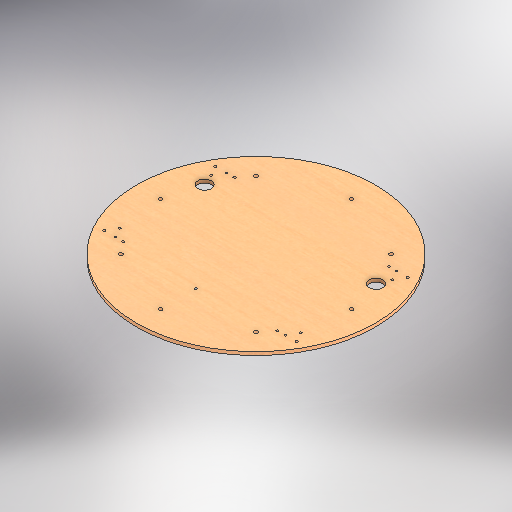
# Autodesk Inventor part: layer3_new
Saved by Autodesk Inventor 2026 (Build 300175050, 175E)
## iProperties
Created: 2025-06-05
Part Number: layer3_new
Material: Generic
Document SubType Name: Modeling
Designer: satom
Density: 1 g/cm^3
Appearance: Default
Author: satom
Autodesk Inventor part; units mm, degrees
ref_plane "YZ Plane" through (0, 0, 0) normal (1, 0, 0) x (0, 1, 0)
ref_plane "XZ Plane" through (0, 0, 0) normal (0, 1, 0) x (-1, 0, 0)
ref_plane "XY Plane" through (0, 0, 0) normal (0, 0, 1) x (1, 0, 0)
sketch "Sketch1" plane through (0, 0, 0) normal (0, 1, 0) x (-1, 0, 0)
  circle A0 centre (0, 0) radius 177
  dimension "d0" = 354
  constraints: 1 centre point, 1 coincident
  measures "d0" diameter of A0
extrude "Extrusion1" add sketch "Sketch1" along normal blind 5
sketch "Sketch2" plane through (0, 5, 0) normal (0, 1, 0) x (1, 0, 0)
  circle A0 centre (-114.3, 82.55) radius 1.7
  line L0 (-177, 0) -> (177, 0) construction
  line L1 (0, 177) -> (0, -177) construction
  circle A1 centre (114.3, 82.55) radius 1.7
  circle A2 centre (-114.3, -82.55) radius 1.7
  circle A3 centre (114.3, -82.55) radius 1.7
  point P0 (0, 0)
  dimension "d3" = 3.4
  dimension "d20" = 82.55
  dimension "d21" = 114.3
  dimension "d24" = 228.6
  dimension "d27" = 165.1
  constraints: 4 centre point, 4 end point, 2 horizontal, 2 vertical, 6 other
  measures "d3" diameter of A0
  measures "d20" distance from line of L0 A0.centre
  measures "d21" distance from line of L1 A0.centre
  measures "d24" distance of A0.centre A1.centre
  measures "d27" distance of A0.centre A2.centre
extrude "Level2 Standoffs" cut sketch "Sketch2" against normal through all
sketch "Sketch3" plane through (0, 5, 0) normal (0, 1, 0) x (1, 0, 0)
  circle A0 centre (-127, 50.8) radius 10.16
  circle A1 centre (127, 50.8) radius 10.16
  circle A2 centre (0, 0) radius 177 construction
  line L0 (0, 177) -> (0, -177) construction
  line L1 (177, 0) -> (-177, 0) construction
  circle A3 centre (0, 0) radius 177 construction
  dimension "d32" = 20.32
  dimension "d33" = 20.32
  dimension "d34" = 127
  dimension "d35" = 127
  dimension "d36" = 50.8
  dimension "d37" = 50.8
  constraints: 5 point on circle, 4 end point, 2 centre point, 1 perpendicular, 1 vertical
  measures "d32" diameter of A0
  measures "d33" diameter of A1
  measures "d34" distance from line of L0 A0.centre
  measures "d35" distance from line of L0 A1.centre
  measures "d36" distance from line of L1 A0.centre
  measures "d37" distance from line of L1 A1.centre
extrude "Wires" cut sketch "Sketch3" against normal through all
sketch "Sketch4" plane through (0, 5, 0) normal (0, 1, 0) x (1, 0, 0)
  line L0 (0, 0) -> (153.2865, -88.5) construction
  circle A0 centre (0, 0) radius 177 construction
  line L1 (-177, 0) -> (177, 0) construction
  circle A1 centre (142.288, -82.15) radius 1.7
  line L2 (142.288, -82.15) -> (134.0391, -77.3875) construction
  line L3 (134.0391, -232.1625) -> (134.0391, -55.1625) construction
  circle A2 centre (134.0391, -67.8625) radius 1.7
  line L4 (268.0782, 0) -> (114.7917, -88.5) construction
  circle A3 centre (125.7902, -82.15) radius 1.7
  circle A4 centre (125.7902, 82.15) radius 1.7
  circle A5 centre (142.288, 82.15) radius 1.7
  circle A6 centre (134.0391, 67.8625) radius 1.7
  line L5 (0, 177) -> (0, -177) construction
  circle A7 centre (-142.288, -82.15) radius 1.7
  circle A8 centre (-134.0391, -67.8625) radius 1.7
  circle A9 centre (-125.7902, -82.15) radius 1.7
  circle A10 centre (-125.7902, 82.15) radius 1.7
  circle A11 centre (-142.288, 82.15) radius 1.7
  circle A12 centre (-134.0391, 67.8625) radius 1.7
  dimension "d40" = 30
  dimension "d41" = 12.7
  dimension "d42" = 9.525
  dimension "d45" = 360
  dimension "d49" = 60
  dimension "d65" = 3.4
  constraints: 12 centre point, 12 end point, 6 point on line, 6 symmetric about line, 5 point on circle, 2 coincident, 1 horizontal, 1 vertical, 30 other
  measures "d40" angle of L0 L1
  measures "d41" distance of L0.end L2.start
  measures "d42" distance of L2.start L2.end
  measures "d65" diameter of A1
extrude "Level4 Standoffs" cut sketch "Sketch4" against normal through all
sketch "Sketch5" plane through (0, 5, 0) normal (0, 1, 0) x (1, 0, 0)
  circle A0 centre (0, -141.44) radius 2.667
  circle A1 centre (0, 0) radius 177 construction
  line L0 (0, -177) -> (89.0082, -177) construction
  circle A2 centre (100.0132, -100.0132) radius 2.667
  circle A3 centre (141.44, 0) radius 2.667
  circle A4 centre (100.0132, 100.0132) radius 2.667
  circle A5 centre (0, 141.44) radius 2.667
  circle A6 centre (-100.0132, 100.0132) radius 2.667
  circle A7 centre (-141.44, 0) radius 2.667
  circle A8 centre (-100.0132, -100.0132) radius 2.667
  dimension "d53" = 5.334
  dimension "d54" = 35.56
  dimension "d57" = 360
  constraints: 8 centre point, 2 end point, 2 horizontal, 1 vertical alignment, 18 other
  measures "d53" diameter of A0
  measures "d54" distance from line of L0 A0.centre
extrude "Zip Ties" cut sketch "Sketch5" against normal through all
sketch "Sketch6" plane through (0, 5, 0) normal (0, 1, 0) x (1, 0, 0)
  circle A0 centre (0, -88.9) radius 1.7
  point P0 (0, 0)
  dimension "d61" = 3.4
  dimension "d62" = 88.9
  constraints: 1 centre point
  measures "d61" diameter of A0
  measures "d62" distance of A0.centre point (0, 0)
extrude "Extrusion6" cut sketch "Sketch6" against normal blind 25.4
equation "\"d0\" = robot_diameter"
equation "\"d1\" = hardboard_thickness"
equation "\"d3\" = m3_clearance"
equation "\"d24\" = 2 * d21"
equation "\"d27\" = 2 * d20"
equation "\"d33\" = d32"
equation "\"d35\" = d34"
equation "\"d37\" = d36"
equation "\"d65\" = m3_clearance"
equation "\"d61\" = m3_clearance"
equation "\"m3_heat_set_insert\" = 4"
equation "\"m3_clearance\" = 3.4"
equation "\"m3_heat_set_depth\" = 7"
equation "\"robot_diameter\" = 354"
equation "\"hardboard_thickness\" = 5"
equation "\"motor_centerline_height\" = 13"
body "Solid1"
